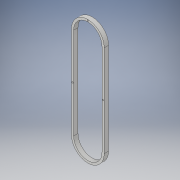
# Autodesk Inventor part: Chain
Saved by Autodesk Inventor 2018 (Build 220112000, 112)
## iProperties
Created: 2017-04-14
Part Number: Chain
Material: Generic
Document SubType Name: Modeling
Designer: Administrator
Density: 1 g/cm^3
Appearance: Default
Author: Administrator
Autodesk Inventor part; units mm, degrees
ref_plane "YZ Plane" through (0, 0, 0) normal (1, 0, 0) x (0, 1, 0)
ref_plane "XZ Plane" through (0, 0, 0) normal (0, 1, 0) x (-1, 0, 0)
ref_plane "XY Plane" through (0, 0, 0) normal (0, 0, 1) x (1, 0, 0)
sketch "Sketch1" plane through (0, 0, 0) normal (0, 0, 1) x (1, 0, 0)
  line L0 (-32.5001, -104.9789) -> (-32.5001, 105.0211)
  line L1 (-32.5001, -104.9789) -> (177.4999, -104.9789) construction
  line L2 (32.5001, -105) -> (32.5001, 105)
  line L3 (32.5001, -105) -> (242.5001, -105) construction
  arc A0 (32.5001, 105) -> (-32.5001, 105.0211) centre (0, 105.0211) ccw
  arc A1 (-32.5001, -104.9789) -> (32.5001, -105) centre (0, -104.9789) ccw
  line L4 (-37.5, -105) -> (-37.5, 105)
  line L5 (-37.5, -105) -> (172.5, -105) construction
  line L6 (37.5, -105) -> (37.5, 105)
  line L7 (37.5, -105) -> (247.5, -105) construction
  arc A2 (-37.5, -105) -> (37.5, -105) centre (0, -105) ccw
  arc A3 (37.5, 105) -> (-37.5, 105) centre (0, 105) ccw
  point P0 (0, 0)
  dimension "d0" = 210
  dimension "d1" = 90
  dimension "d2" = 210
  dimension "d3" = 90
  dimension "d4" = 210
  dimension "d5" = 90
  dimension "d6" = 210
  dimension "d7" = 90
  constraints: 16 end point, 8 point on circle, 4 centre point, 4 horizontal, 4 perpendicular, 4 tangent, 4 vertical
  measures "d0" distance of L0.start L0.end
  measures "d1" angle of L1 L0
  measures "d2" distance of L2.start L2.end
  measures "d3" angle of L3 L2
  measures "d4" distance of L4.start L4.end
  measures "d5" angle of L5 L4
  measures "d6" distance of L6.start L6.end
  measures "d7" angle of L7 L6
extrude "Extrusion1" add sketch "Sketch1" along normal blind 10
sketch "Sketch3" plane through (0, 0, 10) normal (0, 0, 1) x (1, 0, 0)
  circle A0 centre (-35, 0) radius 1.5
  circle A1 centre (0, -140) radius 1.5
  circle A2 centre (35, 0) radius 1.5
  point P0 (0, 0)
  dimension "d11" = 3
  dimension "d12" = 3
  dimension "d13" = 3
  constraints: 3 centre point
  measures "d11" diameter of A0
  measures "d12" diameter of A1
  measures "d13" diameter of A2
hole "Hole1" at (-35, 0, 10) direction (0, 0, -1) diameter 3 end through all
sketch "Sketch5" plane through (0, 0, 10) normal (0, 0, 1) x (1, 0, 0)
  circle A0 centre (35, 0) radius 1.5
  point P0 (0, 0)
  dimension "d31" = 3
  constraints: 1 centre point
  measures "d31" diameter of A0
hole "Hole3" at (35, 0, 10) direction (0, 0, -1) diameter 3 end through all
sketch "Sketch6" plane through (0, 0, 10) normal (0, 0, 1) x (1, 0, 0)
  circle A0 centre (0, 140) radius 1.5
  point P0 (0, 0)
  dimension "d39" = 3
  constraints: 1 centre point
  measures "d39" diameter of A0
hole "Hole4" at (0, 140, 10) direction (0, 0, -1) diameter 3 end through all
body "Solid1"
